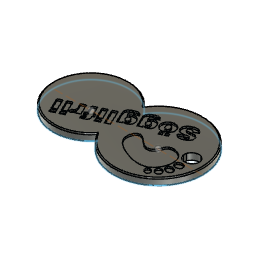
jetton (Autodesk Fusion 360 design; units mm, degrees)
Autodesk Fusion 360 part; units mm, degrees
sketch "Skizze1" plane through (0, 0, 0) normal (0, 0, 1) x (1, 0, 0) in component "Jetton"
  line L0 (-30, 0) -> (16, 0) construction
  arc A0 (-9.3333, -7.2357) -> (-9.3333, 7.2357) centre (2.3, 0) ccw
  arc A1 (-9.3333, 7.2357) -> (-9.3333, -7.2357) centre (-18.4, 0) ccw
  dimension "d1" = 46
  constraint horizontal L0
  constraint coincident L0.start A1
  constraint coincident L0.end A0
  measures "d1" distance of L0.start L0.end
extrude "Extrusion1" add sketch "Skizze1" along normal blind 2 in component "Soegglifrii"
sketch "Skizze1 (2)" plane through (0, 0, 2) normal (0, 0, 1) x (-1, 0, 0) in component "Soegglifrii"
  arc A0 (9.3333, -7.2357) -> (9.3333, 7.2357) centre (18.4, 0) ccw
  arc A1 (9.3333, 7.2357) -> (9.3333, -7.2357) centre (-2.3, 0) ccw
  spline S0 degree 3 poles (3.8178, 1.9102) (3.5968, 1.3606) (3.2317, 0.9957) (2.768, 0.8609) knots 0 0 0 0 1 1 1 1
  spline S1 degree 3 poles (2.768, 0.8609) (2.546, 0.7964) (2.5227, 0.7966) (2.1487, 0.8641) knots 0 0 0 0 1 1 1 1
  spline S2 degree 3 poles (2.1487, 0.8641) (1.793, 0.9283) (1.7386, 0.947) (1.5088, 1.0839) knots 0 0 0 0 1 1 1 1
  spline S3 degree 3 poles (1.5088, 1.0839) (1.2043, 1.2652) (0.6911, 1.6578) (0.1067, 2.1564) knots 0 0 0 0 1 1 1 1
  spline S4 degree 3 poles (0.1067, 2.1564) (-0.3828, 2.5741) (-0.9347, 2.9835) (-1.1982, 3.1246) knots 0 0 0 0 1 1 1 1
  spline S5 degree 3 poles (-1.1982, 3.1246) (-1.4684, 3.2693) (-2.1681, 3.3845) (-2.4684, 3.3338) knots 0 0 0 0 1 1 1 1
  spline S6 degree 3 poles (-2.4684, 3.3338) (-3.403, 3.176) (-4.126, 2.4025) (-4.575, 1.0803) knots 0 0 0 0 1 1 1 1
  spline S7 degree 3 poles (-4.575, 1.0803) (-4.802, 0.4116) (-5.0276, 0.083) (-5.433, -0.17) knots 0 0 0 0 1 1 1 1
  spline S8 degree 3 poles (-5.433, -0.17) (-5.6523, -0.3068) (-6.098, -0.4442) (-6.4138, -0.4725) knots 0 0 0 0 1 1 1 1
  spline S9 degree 3 poles (-6.4138, -0.4725) (-6.7314, -0.5009) (-7.6051, -0.3438) (-7.9502, -0.1962) knots 0 0 0 0 1 1 1 1
  spline S10 degree 3 poles (-7.9502, -0.1962) (-8.2147, -0.0831) (-8.6383, 0.1592) (-8.8491, 0.318) knots 0 0 0 0 1 1 1 1
  spline S11 degree 3 poles (-8.8491, 0.318) (-9.0431, 0.4641) (-9.3576, 0.779) (-9.5305, 1.0002) knots 0 0 0 0 1 1 1 1
  spline S12 degree 3 poles (-9.5305, 1.0002) (-10.0805, 1.7042) (-10.2942, 2.8307) (-10.1263, 4.1408) knots 0 0 0 0 1 1 1 1
  spline S13 degree 3 poles (-10.1263, 4.1408) (-9.9839, 5.2527) (-9.5192, 6.2953) (-8.7458, 7.2384) knots 0 0 0 0 1 1 1 1
  spline S14 degree 3 poles (-8.7458, 7.2384) (-8.1817, 7.9263) (-7.4978, 8.4104) (-6.7883, 8.624) knots 0 0 0 0 1 1 1 1
  spline S15 degree 3 poles (-6.7883, 8.624) (-6.243, 8.7882) (-5.6641, 8.8577) (-4.784, 8.8649) knots 0 0 0 0 1 1 1 1
  spline S16 degree 3 poles (-4.784, 8.8649) (-4.3177, 8.8686) (-4.2229, 8.8584) (-3.425, 8.7181) knots 0 0 0 0 1 1 1 1
  spline S17 degree 3 poles (-3.425, 8.7181) (-2.7951, 8.6073) (-2.4453, 8.5299) (-2.1082, 8.4265) knots 0 0 0 0 1 1 1 1
  spline S18 degree 3 poles (-2.1082, 8.4265) (0.2054, 7.7175) (2.1321, 6.6537) (3.1695, 5.5125) knots 0 0 0 0 1 1 1 1
  spline S19 degree 3 poles (3.1695, 5.5125) (3.7181, 4.909) (3.9826, 4.3536) (4.034, 3.6973) knots 0 0 0 0 1 1 1 1
  spline S20 degree 3 poles (4.034, 3.6973) (4.0857, 3.036) (4.0062, 2.3788) (3.8178, 1.9102) knots 0 0 0 0 1 1 1 1
  spline S21 degree 3 poles (-7.6486, 8.7634) (-7.7517, 8.6171) (-7.9571, 8.4884) (-8.1267, 8.4637) knots 0 0 0 0 1 1 1 1
  spline S22 degree 3 poles (-8.1267, 8.4637) (-8.3425, 8.4324) (-8.7174, 8.5397) (-8.8997, 8.685) knots 0 0 0 0 1 1 1 1
  spline S23 degree 3 poles (-8.8997, 8.685) (-9.1079, 8.8509) (-9.3002, 9.16) (-9.3327, 9.3808) knots 0 0 0 0 1 1 1 1
  spline S24 degree 3 poles (-9.3327, 9.3808) (-9.3895, 9.7666) (-9.187, 10.1205) (-8.8496, 10.2251) knots 0 0 0 0 1 1 1 1
  spline S25 degree 3 poles (-8.8496, 10.2251) (-8.6006, 10.3023) (-8.2581, 10.2397) (-8.0183, 10.0733) knots 0 0 0 0 1 1 1 1
  spline S26 degree 3 poles (-8.0183, 10.0733) (-7.8212, 9.9364) (-7.6298, 9.6791) (-7.5629, 9.4609) knots 0 0 0 0 1 1 1 1
  spline S27 degree 3 poles (-7.5629, 9.4609) (-7.4971, 9.2464) (-7.537, 8.9217) (-7.6486, 8.7634) knots 0 0 0 0 1 1 1 1
  spline S28 degree 3 poles (-9.788, -1.2423) (-10.1708, -2.4549) (-11.5903, -3.1545) (-12.7794, -2.7166) knots 0 0 0 0 1 1 1 1
  spline S29 degree 3 poles (-12.7794, -2.7166) (-13.8536, -2.321) (-14.3715, -1.1577) (-13.9392, -0.1117) knots 0 0 0 0 1 1 1 1
  spline S30 degree 3 poles (-13.9392, -0.1117) (-13.6199, 0.6605) (-12.8907, 1.1973) (-12.006, 1.3112) knots 0 0 0 0 1 1 1 1
  spline S31 degree 3 poles (-12.006, 1.3112) (-11.7955, 1.3384) (-11.6808, 1.3318) (-11.3617, 1.2744) knots 0 0 0 0 1 1 1 1
  spline S32 degree 3 poles (-11.3617, 1.2744) (-11.0145, 1.2119) (-10.9463, 1.1891) (-10.7143, 1.0581) knots 0 0 0 0 1 1 1 1
  spline S33 degree 3 poles (-10.7143, 1.0581) (-10.1329, 0.7298) (-9.7797, 0.2096) (-9.713, -0.4165) knots 0 0 0 0 1 1 1 1
  spline S34 degree 3 poles (-9.713, -0.4165) (-9.6819, -0.7085) (-9.7071, -0.9861) (-9.788, -1.2423) knots 0 0 0 0 1 1 1 1
  spline S35 degree 3 poles (-9.2784, 7.3236) (-9.4039, 7.0423) (-9.7091, 6.7889) (-9.9678, 6.7514) knots 0 0 0 0 1 1 1 1
  spline S36 degree 3 poles (-9.9678, 6.7514) (-10.1764, 6.7211) (-10.5219, 6.8221) (-10.74, 6.9772) knots 0 0 0 0 1 1 1 1
  spline S37 degree 3 poles (-10.74, 6.9772) (-11.1577, 7.2742) (-11.3399, 7.6535) (-11.2633, 8.0662) knots 0 0 0 0 1 1 1 1
  spline S38 degree 3 poles (-11.2633, 8.0662) (-11.1964, 8.427) (-10.989, 8.6785) (-10.6565, 8.8025) knots 0 0 0 0 1 1 1 1
  spline S39 degree 3 poles (-10.6565, 8.8025) (-10.5132, 8.856) (-10.4554, 8.8582) (-10.2317, 8.8187) knots 0 0 0 0 1 1 1 1
  spline S40 degree 3 poles (-10.2317, 8.8187) (-10.0013, 8.7781) (-9.9483, 8.7556) (-9.7505, 8.6142) knots 0 0 0 0 1 1 1 1
  spline S41 degree 3 poles (-9.7505, 8.6142) (-9.4954, 8.4318) (-9.3042, 8.1865) (-9.2399, 7.9592) knots 0 0 0 0 1 1 1 1
  spline S42 degree 3 poles (-9.2399, 7.9592) (-9.1876, 7.7744) (-9.205, 7.4883) (-9.2784, 7.3236) knots 0 0 0 0 1 1 1 1
  spline S43 degree 3 poles (-10.7805, 2.684) (-10.9359, 2.3892) (-11.4163, 2.1453) (-11.8919, 2.1199) knots 0 0 0 0 1 1 1 1
  spline S44 degree 3 poles (-11.8919, 2.1199) (-12.6537, 2.0792) (-13.2092, 2.668) (-13.0831, 3.3826) knots 0 0 0 0 1 1 1 1
  spline S45 degree 3 poles (-13.0831, 3.3826) (-13.0104, 3.7949) (-12.7588, 4.0358) (-12.2586, 4.1719) knots 0 0 0 0 1 1 1 1
  spline S46 degree 3 poles (-12.2586, 4.1719) (-11.5077, 4.3762) (-10.8778, 4.0731) (-10.7094, 3.4265) knots 0 0 0 0 1 1 1 1
  spline S47 degree 3 poles (-10.7094, 3.4265) (-10.6484, 3.1923) (-10.6786, 2.8776) (-10.7805, 2.684) knots 0 0 0 0 1 1 1 1
  spline S48 degree 3 poles (-10.3383, 5.1823) (-10.4851, 4.9037) (-10.8341, 4.7022) (-11.2067, 4.6811) knots 0 0 0 0 1 1 1 1
  spline S49 degree 3 poles (-11.2067, 4.6811) (-11.7056, 4.6528) (-12.2475, 4.8941) (-12.4849, 5.2503) knots 0 0 0 0 1 1 1 1
  spline S50 degree 3 poles (-12.4849, 5.2503) (-12.7923, 5.7113) (-12.6998, 6.2475) (-12.2648, 6.5264) knots 0 0 0 0 1 1 1 1
  spline S51 degree 3 poles (-12.2648, 6.5264) (-12.0048, 6.6932) (-11.8258, 6.7247) (-11.4377, 6.6724) knots 0 0 0 0 1 1 1 1
  spline S52 degree 3 poles (-11.4377, 6.6724) (-11.058, 6.6211) (-10.7793, 6.5018) (-10.5716, 6.3014) knots 0 0 0 0 1 1 1 1
  spline S53 degree 3 poles (-10.5716, 6.3014) (-10.2588, 5.9997) (-10.1592, 5.5223) (-10.3383, 5.1823) knots 0 0 0 0 1 1 1 1
extrude "Extrusion5" cut sketch "Skizze1 (2)" against normal through all contours S28 S29 S30 S31 S32 S33 S34 in component "Soegglifrii"
extrude "Extrusion6" cut sketch "Skizze1 (2)" against normal blind 0.5 contours S0 S1 S2 S3 S4 S5 S6 S7 S8 S9 S10 S11 S12 S13 S14 S15 S16 S17 S18 S19 S20 | S21 S22 S23 S24 S25 S26 S27 | S35 S36 S37 S38 S39 S40 S41 S42 | S43 S44 S45 S46 S47 | S48 S49 S50 S51 S52 S53 in component "Soegglifrii"
sketch "Skizze2" plane through (0, 0, 2) normal (0, 0, 1) x (1, 0, 0) in component "Soegglifrii"
  line L0 (4.7867, 11.9698) -> (-27.4867, -3.1215) construction
  line L1 (-27.4867, -3.1215) -> (-24.4764, -9.5592) construction
  line L2 (-24.4764, -9.5592) -> (7.797, 5.532) construction
  line L3 (7.797, 5.532) -> (4.7867, 11.9698) construction
  dimension "d17" = 5
  text T0 "Sögglifrii" font "Arial Black" height 5 align left top in box 35.6275 x 7.1068 at (4.7867, 11.9698) x (-0.905857, -0.423584) y (0.423584, -0.905857) spacing 1 kerned
extrude "Extrusion8" cut sketch "Skizze2" against normal blind 0.5 text T0 in component "Soegglifrii"
fillet "Abrundung1" radius 0.3 2 edges at (16, 0, 2) (-30, 0, 2) in component "Soegglifrii"
component "Jetton" placed x (1, 0, 0) y (0, 1, 0) z (0, 0, 1) at (0, 0, 0)
component "Soegglifrii" placed x (1, 0, 0) y (0, 1, 0) z (0, 0, 1) at (0, 0, 0)
